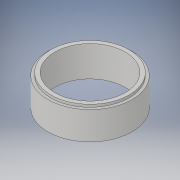
# Autodesk Inventor part: Retainer
Saved by Autodesk Inventor 2017 (Build 210142000, 142)
## iProperties
Created: 2016-07-19
Part Number: Retainer
Material: Generic
Document SubType Name: Modeling
Designer: Bill
Density: 1 g/cm^3
Appearance: Default
Author: Bill
Autodesk Inventor part; units mm, degrees
ref_plane "YZ Plane" through (0, 0, 0) normal (1, 0, 0) x (0, 1, 0)
ref_plane "XZ Plane" through (0, 0, 0) normal (0, 1, 0) x (-1, 0, 0)
ref_plane "XY Plane" through (0, 0, 0) normal (0, 0, 1) x (1, 0, 0)
sketch "Sketch1" plane through (0, 0, 0) normal (0, 0, 1) x (1, 0, 0)
  line L0 (-80.0608, 24.4238) -> (-88.9, 24.4238)
  line L1 (-88.9, 24.4238) -> (-88.9, 18.4802)
  line L2 (-88.9, 18.4802) -> (-95.25, 18.4802)
  line L3 (-95.25, 18.4802) -> (-95.25, -45.0198)
  line L4 (-95.25, -45.0198) -> (-80.0608, -45.0198)
  line L5 (-80.0608, -45.0198) -> (-80.0608, 24.4238)
  line L6 (0, -58.9086) -> (0, 38.3125) projected
  point P0 (0, 0)
  dimension "d0" = 8.8392
  dimension "d1" = 6.35
  dimension "d2" = 5.9436
  dimension "d3" = 63.5
  dimension "d4" = 80.0608
  dimension "d6" = 95.25
  constraints: 12 end point, 5 perpendicular, 1 horizontal
  measures "d0" distance of L0.start L0.end
  measures "d1" distance of L1.end L2.end
  measures "d2" distance of L0.end L1.end
  measures "d3" distance of L2.end L3.end
  measures "d4" horizontal distance of point (0, 0) L4.end
  measures "d6" distance between parallel lines of L6 L3
revolve "Revolution1" add sketch "Sketch1" angle 360 about axis through (0, -10, 0) along (0, 1, 0)
body "Solid1"
